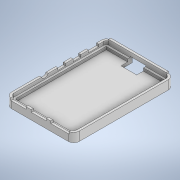
# Autodesk Inventor part: piholder-proto-v5
Saved by Autodesk Inventor 2022 (Build 260153000, 153)
## iProperties
Created: 2021-07-08
Part Number: piholder-proto-v5
Material: Generic
Document SubType Name: Modeling
Designer: dncob
Density: 1 g/cm^3
Appearance: Default
Author: dncob
Autodesk Inventor part; units mm, degrees
ref_plane "YZ Plane" through (0, 0, 0) normal (1, 0, 0) x (0, 1, 0)
ref_plane "XZ Plane" through (0, 0, 0) normal (0, 1, 0) x (-1, 0, 0)
ref_plane "XY Plane" through (0, 0, 0) normal (0, 0, 1) x (1, 0, 0)
sketch "Sketch1" plane through (0, 0, 0) normal (0, 1, 0) x (-1, 0, 0)
  line L0 (-25.25, 42.75) -> (25.25, 42.75)
  line L1 (28.25, 39.75) -> (28.25, -40.75)
  line L2 (26.25, -42.75) -> (-25.25, -42.75)
  line L3 (-28.25, -39.75) -> (-28.25, 39.75)
  line L4 (-28.25, 42.75) -> (28.25, -42.75) construction
  line L5 (28.25, 42.75) -> (-28.25, -42.75) construction
  arc A0 (26.25, -42.75) -> (28.25, -40.75) centre (26.25, -40.75) ccw
  arc A1 (-28.25, -39.75) -> (-25.25, -42.75) centre (-25.25, -39.75) ccw
  arc A2 (-25.25, 42.75) -> (-28.25, 39.75) centre (-25.25, 39.75) ccw
  arc A3 (28.25, 39.75) -> (25.25, 42.75) centre (25.25, 39.75) ccw
  line L6 (30.25, -40.75) -> (30.25, 39.75)
  arc A4 (30.25, 39.75) -> (25.25, 44.75) centre (25.25, 39.75) ccw
  line L7 (25.25, 44.75) -> (-25.25, 44.75)
  arc A5 (-25.25, 44.75) -> (-30.25, 39.75) centre (-25.25, 39.75) ccw
  line L8 (-30.25, 39.75) -> (-30.25, -39.75)
  arc A6 (-30.25, -39.75) -> (-25.25, -44.75) centre (-25.25, -39.75) ccw
  line L9 (-25.25, -44.75) -> (26.25, -44.75)
  arc A7 (26.25, -44.75) -> (30.25, -40.75) centre (26.25, -40.75) ccw
  point P0 (0, 0)
  dimension "d0" = 56.5
  dimension "d1" = 85.5
  dimension "d2" = 2
  dimension "d3" = 3
  dimension "d4" = 2
  constraints: 20 end point, 16 point on circle, 8 centre point, 8 point on line, 8 tangent, 4 parallel, 2 equal radius, 2 midpoint, 2 perpendicular, 1 horizontal, 7 other
  measures "d0" distance of L4.end L5.end
  measures "d1" distance of L5.start L4.end
  measures "d2" radius of A0
  measures "d3" radius of A1
  measures "d4" distance between parallel lines of L1 L6
extrude "Extrusion1" add sketch "Sketch1" along normal blind 3
sketch "Sketch2" plane through (0, 0, 0) normal (0, -1, 0) x (1, 0, 0)
  arc A0 (-25.25, 44.75) -> (-30.25, 39.75) centre (-25.25, 39.75) ccw projected
  line L0 (-25.25, 44.75) -> (25.25, 44.75) projected
  arc A1 (30.25, 39.75) -> (25.25, 44.75) centre (25.25, 39.75) ccw projected
  line L1 (30.25, 39.75) -> (30.25, -39.75) projected
  arc A2 (25.25, -44.75) -> (30.25, -39.75) centre (25.25, -39.75) ccw projected
  line L2 (25.25, -44.75) -> (-26.25, -44.75) projected
  arc A3 (-30.25, -40.75) -> (-26.25, -44.75) centre (-26.25, -40.75) ccw projected
  line L3 (-30.25, -40.75) -> (-30.25, 39.75) projected
  line L4 (-26.25, -44.75) -> (25.25, -44.75)
  line L5 (30.25, -39.75) -> (30.25, 39.75)
  line L6 (25.25, 44.75) -> (-25.25, 44.75)
  line L7 (-30.25, 39.75) -> (-30.25, -40.75)
  line L8 (-30, -44.5) -> (30, 44.5) construction
  line L9 (30, -44.5) -> (-30, 44.5) construction
  arc A4 (-25.25, 44.75) -> (-30.25, 39.75) centre (-25.25, 39.75) ccw
  arc A5 (30.25, 39.75) -> (25.25, 44.75) centre (25.25, 39.75) ccw
  arc A6 (25.25, -42.75) -> (28.25, -39.75) centre (25.25, -39.75) ccw projected
  arc A7 (25.25, -44.75) -> (30.25, -39.75) centre (25.25, -39.75) ccw
  arc A8 (-30.25, -40.75) -> (-26.25, -44.75) centre (-26.25, -40.75) ccw
  line L10 (25.25, 40.75) -> (-25.25, 40.75)
  arc A9 (-25.25, 40.75) -> (-26.25, 39.75) centre (-25.25, 39.75) ccw
  line L11 (-26.25, 39.75) -> (-26.25, -40.75)
  line L12 (-26.25, -40.75) -> (25.25, -40.75)
  arc A10 (25.25, -40.75) -> (26.25, -39.75) centre (25.25, -39.75) ccw
  line L13 (26.25, -39.75) -> (26.25, 39.75)
  arc A11 (26.25, 39.75) -> (25.25, 40.75) centre (25.25, 39.75) ccw
  point P0 (0, 0)
  point P1 (-26.25, -40.75)
  dimension "d12" = 4
  constraints: 21 end point, 14 point on circle, 7 centre point, 4 coincident, 4 concentric, 4 point on line, 2 collinear, 2 midpoint, 2 parallel, 1 horizontal, 1 perpendicular, 11 other
  measures "d12" distance between parallel lines of L10 L0
extrude "Extrusion2" add sketch "Sketch2" along normal blind 2.5
sketch "Sketch3" plane through (25.25, 3, -44.75) normal (0, 0, -1) x (-1, 0, 0)
  line L0 (51.5, -5.5) -> (51.5, 0) projected
  line L1 (51.5, 0) -> (0, 0)
  line L2 (0, 0) -> (0, 1.5)
  line L3 (0, 1.5) -> (51.5, 1.5)
  line L4 (51.5, 1.5) -> (51.5, 0)
  point P0 (25.25, -3)
  dimension "d9" = 1.5
  constraints: 8 end point, 2 parallel, 1 coincident, 1 horizontal, 1 perpendicular
  measures "d9" distance between parallel lines of L1 L3
extrude "Extrusion3" add sketch "Sketch3" against normal blind 2
sketch "Sketch4" plane through (0, -2.5, 0) normal (0, -1, 0) x (1, 0, 0)
  line L0 (25.25, 44.75) -> (-25.25, 44.75)
  line L1 (-30.25, 39.75) -> (-30.25, -40.75)
  line L2 (-26.25, -44.75) -> (25.25, -44.75)
  line L3 (30.25, -39.75) -> (30.25, 39.75)
  line L4 (30, 44.5) -> (-30, -44.5) construction
  line L5 (-30, 44.5) -> (30, -44.5) construction
  line L6 (-26.25, -44.75) -> (25.25, -44.75) projected
  line L7 (-30.25, 39.75) -> (-30.25, -40.75) projected
  arc A0 (25.25, -44.75) -> (30.25, -39.75) centre (25.25, -39.75) ccw projected
  arc A1 (-30.25, -40.75) -> (-26.25, -44.75) centre (-26.25, -40.75) ccw projected
  arc A2 (-25.25, 44.75) -> (-30.25, 39.75) centre (-25.25, 39.75) ccw projected
  arc A3 (30.25, 39.75) -> (25.25, 44.75) centre (25.25, 39.75) ccw projected
  arc A4 (25.25, -44.75) -> (30.25, -39.75) centre (25.25, -39.75) ccw
  line L8 (25.25, -40.75) -> (-26.25, -40.75) projected
  arc A5 (-30.25, -40.75) -> (-26.25, -44.75) centre (-26.25, -40.75) ccw
  arc A6 (-25.25, 44.75) -> (-30.25, 39.75) centre (-25.25, 39.75) ccw
  arc A7 (30.25, 39.75) -> (25.25, 44.75) centre (25.25, 39.75) ccw
  line L9 (25.25, 44.75) -> (-25.25, 44.75) projected
  point P0 (0, 0)
  point P1 (-30.25, 39.75)
  point P2 (-30.25, -40.75)
  point P3 (25.25, -44.75)
  constraints: 13 end point, 10 point on circle, 4 centre point, 4 coincident, 4 concentric, 4 point on line, 3 collinear, 2 midpoint, 2 parallel, 1 horizontal, 1 perpendicular
extrude "Extrusion4" add sketch "Sketch4" along normal blind 2.5
sketch "Sketch5" plane through (25.25, 4.5, -44.75) normal (0, 0, -1) x (-1, 0, 0)
  line L0 (51.5, -9.5) -> (0, -9.5) projected
  line L1 (18.25, -9.5) -> (32.25, -9.5)
  line L2 (32.25, -9.5) -> (32.25, -3.5)
  line L3 (32.25, -3.5) -> (18.25, -3.5)
  line L4 (18.25, -3.5) -> (18.25, -9.5)
  line L5 (18.25, -9.5) -> (32.25, -3.5) construction
  line L6 (32.25, -9.5) -> (18.25, -3.5) construction
  point P0 (25.25, -4.5)
  point P1 (25.25, -6.5)
  dimension "d16" = 14
  dimension "d17" = 0
  dimension "d18" = 6
  constraints: 12 end point, 2 midpoint, 2 parallel, 1 horizontal, 1 perpendicular, 1 vertical alignment
  measures "d16" distance of L2.end L3.end
  measures "d17" distance between parallel lines of L0 L1
  measures "d18" distance between parallel lines of L1 L3
extrude "Extrusion5" cut sketch "Sketch5" against normal blind 10
sketch "Sketch6" plane through (-30.25, 3, -40.75) normal (-1, 0, 0) x (0, 0, 1)
  line L0 (1, 0) -> (80.5, 0) projected
  line L1 (4.6696, 0) -> (13.8622, 0)
  line L2 (13.8622, 0) -> (13.8622, -2)
  line L3 (13.8622, -2) -> (4.6696, -2)
  line L4 (4.6696, -2) -> (4.6696, 0)
  line L5 (20.7687, 0) -> (27.5371, 0)
  line L6 (27.5371, 0) -> (27.5371, -2)
  line L7 (27.5371, -2) -> (20.7687, -2)
  line L8 (20.7687, -2) -> (20.7687, 0)
  line L9 (34.3481, 0) -> (41.1165, 0)
  line L10 (41.1165, 0) -> (41.1165, -2)
  line L11 (41.1165, -2) -> (34.3481, -2)
  line L12 (34.3481, -2) -> (34.3481, 0)
  arc A0 (49.8136, 0) -> (55.8136, 0) centre (52.8136, 1.25) ccw
  line L13 (-2, 1.5) -> (-2, 0) projected
  line L14 (80.5, -8) -> (0, -8) projected
  line L15 (49.8136, 0) -> (55.8136, 0)
  point P0 (40.75, -3)
  dimension "d21" = 6.6696
  dimension "d22" = 9.1926
  dimension "d23" = 22.7687
  dimension "d25" = 6.7684
  dimension "d26" = 6.7684
  dimension "d27" = 36.3481
  dimension "d28" = 51.8136
  dimension "d29" = 6
  dimension "d30" = 2
  constraints: 26 end point, 6 parallel, 5 point on line, 3 horizontal, 3 perpendicular, 2 collinear, 2 point on circle, 1 centre point, 1 tangent
  measures "d21" distance between parallel lines of L4 L13
  measures "d22" distance of L2.end L3.end
  measures "d23" distance between parallel lines of L8 L13
  measures "d25" distance of L6.end L7.end
  measures "d26" distance of L10.end L11.end
  measures "d27" distance from line of L12 L13.start
  measures "d28" horizontal distance of L15.start L13.start
  measures "d29" distance of L15.end L15.start
  measures "d30" distance of L9.end L10.end
extrude "Extrusion6" cut sketch "Sketch6" against normal up to surface (2 mm away)
sketch "Sketch7" plane through (-25.25, 3, 44.75) normal (0, 0, 1) x (1, 0, 0)
  line L0 (50.5, 0) -> (0, 0) projected
  line L1 (-0.7188, 0) -> (12.8798, 0)
  line L2 (12.8798, 0) -> (12.8798, -2)
  line L3 (12.8798, -2) -> (-0.7188, -2)
  line L4 (-0.7188, -2) -> (-0.7188, 0)
  line L5 (17.4418, 0) -> (31.0404, 0)
  line L6 (31.0404, 0) -> (31.0404, -2)
  line L7 (31.0404, -2) -> (17.4418, -2)
  line L8 (17.4418, -2) -> (17.4418, 0)
  line L9 (34.977, 0) -> (51.34, 0)
  line L10 (51.34, 0) -> (51.34, -2)
  line L11 (51.34, -2) -> (34.977, -2)
  line L12 (34.977, -2) -> (34.977, 0)
  line L13 (-3, -3) -> (-3, 0) projected
  point P0 (25.25, -3)
  dimension "d33" = 2
  dimension "d34" = 2.2812
  dimension "d35" = 13.5986
  dimension "d36" = 20.4418
  dimension "d37" = 13.5986
  dimension "d38" = 37.977
  dimension "d39" = 16.363
  constraints: 24 end point, 6 parallel, 5 point on line, 3 horizontal, 3 perpendicular
  measures "d33" distance of L9.end L10.end
  measures "d34" distance between parallel lines of L4 L13
  measures "d35" distance of L1.start L1.end
  measures "d36" distance between parallel lines of L8 L13
  measures "d37" distance of L5.start L5.end
  measures "d38" distance between parallel lines of L12 L13
  measures "d39" distance of L9.start L9.end
extrude "Extrusion7" cut sketch "Sketch7" against normal blind 5
body "Solid1"
